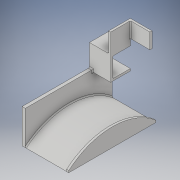
# Autodesk Inventor part: headphonesDeskHanger
Saved by Autodesk Inventor 2017 (Build 210142000, 142)
## iProperties
Created: 2017-01-28
Part Number: headphonesDeskHanger
Material: Generic
Document SubType Name: Modeling
Designer: jjaken
Density: 1 g/cm^3
Appearance: Default
Author: jjaken
Autodesk Inventor part; units mm, degrees
ref_plane "YZ Plane" through (0, 0, 0) normal (1, 0, 0) x (0, 1, 0)
ref_plane "XZ Plane" through (0, 0, 0) normal (0, 1, 0) x (-1, 0, 0)
ref_plane "XY Plane" through (0, 0, 0) normal (0, 0, 1) x (1, 0, 0)
sketch "Sketch1" plane through (0, 0, 0) normal (1, 0, 0) x (0, 1, 0)
  line L0 (9.25, -16.5) -> (11.25, -16.5)
  line L1 (11.25, -16.5) -> (11.25, 2)
  line L2 (11.25, 2) -> (-11.25, 2)
  line L3 (-11.25, 2) -> (-11.25, -16.5)
  line L4 (-11.25, -16.5) -> (-9.25, -16.5)
  line L5 (-9.25, -16.5) -> (-9.25, 0)
  line L6 (-9.25, 0) -> (9.25, 0)
  line L7 (9.25, 0) -> (9.25, -16.5)
  point P0 (0, 0)
  point P1 (0, 0)
  point P2 (10.25, -16.5)
  point P3 (-10.25, -16.5)
  dimension "d0" = 18.5
  dimension "d1" = 2
  dimension "d2" = 2
  dimension "d3" = 18.5
  constraints: 16 end point, 5 perpendicular, 3 midpoint, 2 point on line, 1 coincident, 1 collinear, 1 horizontal alignment, 1 vertical
  measures "d0" distance between parallel lines of L5 L7
  measures "d1" distance of L0.start L0.end
  measures "d2" distance between parallel lines of L6 L2
  measures "d3" distance of L0.end L1.end
extrude "Extrusion1" add sketch "Sketch1" along normal blind 20
sketch "Sketch2" plane through (20, 0, 0) normal (1, 0, 0) x (0, 0, -1)
  line L0 (16.5, 9.25) -> (16.5, 11.25) projected
  line L1 (16.5, 11.25) -> (-2, 11.25) projected
  line L2 (-2, 11.25) -> (-2, -11.25) projected
  line L3 (-2, -11.25) -> (16.5, -11.25) projected
  line L4 (16.5, -11.25) -> (16.5, -9.25) projected
  line L5 (16.5, -9.25) -> (0, -9.25) projected
  line L6 (0, -9.25) -> (0, 9.25) projected
  line L7 (0, 9.25) -> (16.5, 9.25) projected
  line L8 (16.5, 9.25) -> (16.5, 11.25) projected
  line L9 (16.5, 11.25) -> (-2, 11.25)
  line L10 (-2, 11.25) -> (-2, 29.75)
  line L11 (-2, 29.75) -> (16.5, 29.75)
  line L12 (16.5, 29.75) -> (16.5, 11.25)
  point P0 (0, 0)
  dimension "d6" = 18.5
  constraints: 8 end point, 2 parallel, 1 horizontal, 1 perpendicular
  measures "d6" distance between parallel lines of L1 L11
extrude "Extrusion2" add sketch "Sketch2" against normal blind 2 contours L1 L10 L11 L12
sketch "Sketch3" plane through (20, 0, 0) normal (1, 0, 0) x (0, 0, -1)
  line L0 (16.5, 9.25) -> (16.5, 29.75) projected
  line L1 (16.5, 29.75) -> (-2, 29.75) projected
  line L2 (-2, 29.75) -> (-2, -11.25) projected
  line L3 (-2, -11.25) -> (16.5, -11.25) projected
  line L4 (16.5, -11.25) -> (16.5, -9.25) projected
  line L5 (16.5, -9.25) -> (0, -9.25) projected
  line L6 (0, -9.25) -> (0, 9.25) projected
  line L7 (0, 9.25) -> (16.5, 9.25) projected
  line L8 (16.5, 29.75) -> (16.5, 15.25)
  line L9 (16.5, 9.25) -> (16.5, 29.75) projected
  line L10 (16.5, 15.25) -> (18.5, 15.25)
  line L11 (18.5, 15.25) -> (18.5, 29.75)
  line L12 (18.5, 29.75) -> (16.5, 29.75)
  point P0 (0, 0)
  dimension "d9" = 6
  dimension "d10" = 2
  constraints: 8 end point, 2 perpendicular, 1 horizontal, 1 point on line
  measures "d9" distance from line of L0.start L10
  measures "d10" distance of L11.end L0.end
extrude "Extrusion3" add sketch "Sketch3" along normal blind 18.5 and the other way blind 2 contours L0 L12 L11 L10
sketch "Sketch4" plane through (0, 0, 0) normal (-1, 0, 0) x (0, 0, 1)
  line L0 (-16.5, 9.25) -> (-16.5, 11.25) projected
  line L1 (0, 9.25) -> (-16.5, 9.25) projected
  line L2 (0, -9.25) -> (0, 9.25) projected
  line L3 (-16.5, -9.25) -> (0, -9.25) projected
  line L4 (-16.5, -11.25) -> (-16.5, -9.25) projected
  line L5 (2, -11.25) -> (-16.5, -11.25) projected
  line L6 (2, 11.25) -> (2, -11.25) projected
  line L7 (-16.5, 11.25) -> (2, 11.25) projected
  line L8 (-16.5, -9.25) -> (0, -9.25) projected
  line L9 (-16.5, -9.25) -> (65.5, -9.25)
  line L10 (65.5, -9.25) -> (65.5, -41.25)
  line L11 (65.5, -41.25) -> (-16.5, -41.25)
  line L12 (-16.5, -41.25) -> (-16.5, -9.25)
  point P0 (0, 0)
  dimension "d15" = 82
  dimension "d16" = 30
  constraints: 8 end point, 2 parallel, 1 horizontal, 1 perpendicular
  measures "d15" distance of L10.end L11.end
  measures "d16" distance between parallel lines of L11 L5
extrude "Extrusion4" add sketch "Sketch4" against normal blind 3 contours L9 L6 L5 L4 L3 | L9 L10 L11 L12 L5 L6
sketch "Sketch5" plane through (3, 0, 0) normal (1, 0, 0) x (0, 0, -1)
  line L0 (-2, -9.25) -> (-2, -11.25) projected
  line L1 (-2, -9.25) -> (-65.5, -9.25) projected
  line L2 (-65.5, -9.25) -> (-65.5, -41.25) projected
  line L3 (-65.5, -41.25) -> (16.5, -41.25) projected
  line L4 (16.5, -41.25) -> (16.5, -11.25) projected
  line L5 (-2, -11.25) -> (16.5, -11.25) projected
  arc A0 (16.5, -41.25) -> (-65.5, -41.25) centre (-24.5, -89.7833) ccw
  point P0 (0, 0)
  dimension "d20" = 15
  constraints: 2 point on circle, 1 centre point
  measures "d20" distance edge to line of A0 L5
extrude "Extrusion5" add sketch "Sketch5" along normal blind 39 contours A0 L3
sketch "Sketch7" plane through (42, 0, 0) normal (1, 0, 0) x (0, 0, -1)
  line L0 (-65.5, -41.25) -> (16.5, -41.25) projected
  arc A0 (16.5, -41.25) -> (-65.5, -41.25) centre (-24.5, -89.7833) ccw projected
  line L1 (-67.5, -41.25) -> (18.5, -41.25)
  arc A1 (18.5, -41.25) -> (-67.5, -41.25) centre (-24.5, -87.1324) ccw
  point P0 (0, 0)
  dimension "d33" = 2
  dimension "d34" = 2
  dimension "d35" = 2
  constraints: 2 end point, 2 point on circle, 1 centre point, 1 collinear, 1 horizontal
  measures "d33" distance of L0.start L1.start
  measures "d34" distance of L0.end L1.end
extrude "Extrusion6" add sketch "Sketch7" along normal blind 2
sketch "Sketch8" plane through (44, 0, 0) normal (1, 0, 0) x (0, 0, -1)
  arc A0 (16.5, -41.25) -> (-65.5, -41.25) centre (-24.5, -89.7833) ccw projected
  line L0 (16.5, -41.25) -> (16.5, -11.25) projected
  line L1 (-2, -11.25) -> (16.5, -11.25) projected
  line L2 (-2, -9.25) -> (-2, -11.25) projected
  line L3 (-2, -9.25) -> (-65.5, -9.25) projected
  line L4 (-65.5, -9.25) -> (-65.5, -41.25) projected
  line L5 (-67.5, -41.25) -> (18.5, -41.25) projected
  arc A1 (18.5, -41.25) -> (-67.5, -41.25) centre (-24.5, -87.1324) ccw projected
  arc A2 (18.5, -41.25) -> (-67.5, -41.25) centre (-24.5, -87.1324) ccw projected
  line L6 (-67.5, -41.25) -> (-65.5, -41.25)
  line L7 (-65.5, -41.25) -> (-65.5, -39.4544)
  line L8 (-65.5, -39.4544) -> (-67.5, -39.4544)
  line L9 (-67.5, -39.4544) -> (-67.5, -41.25)
  line L10 (16.5, -41.25) -> (18.5, -41.25) projected
  line L11 (16.5, -9.25) -> (16.5, -41.25) projected
  line L12 (18.5, -41.25) -> (16.5, -41.25)
  line L13 (16.5, -41.25) -> (16.5, -39.4544)
  line L14 (16.5, -39.4544) -> (18.5, -39.4544)
  line L15 (18.5, -39.4544) -> (18.5, -41.25)
  point P0 (0, 0)
  constraints: 16 end point, 4 parallel, 3 point on circle, 2 horizontal, 2 perpendicular, 1 point on line
extrude "Extrusion7" cut sketch "Sketch8" against normal up to surface (2 mm away) contours L0 A1 L5 | L5 A1 L4
fillet "Fillet1" radius 1 9 edges at (3, -26.25, 24.5) (20, 22.5, -16.5) (1.5, -9.25, 2) (3, -10.25, 2) (3, -11.25, -7.25) (10, 9.25, 0) (10, -9.25, 0) (18, 11.25, -7.25) (19, 15.25, -16.5)
equation "\"d2\" = d1"
equation "\"d3\" = d0"
equation "\"d34\" = d33"
body "Solid1"
